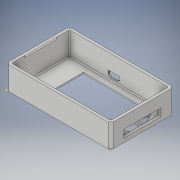
# Autodesk Inventor part: Top
Saved by Autodesk Inventor 2019 (Build 230136000, 136)
## iProperties
Created: 2021-04-22
Part Number: Top
Material: Všeobecné
Document SubType Name: Modeling
Designer: miko flosso
Density: 1 g/cm^3
Appearance: Výchozí
Author: miko flosso
Autodesk Inventor part; units mm, degrees
sketch "Náčrt1" plane through (0, 0, 0) normal (0, 1, 0) x (-1, 0, 0)
  line L0 (0, 0) -> (-81, 0)
  line L1 (-81, 0) -> (-81, -49)
  line L2 (-81, -49) -> (0, -49)
  line L3 (0, -49) -> (0, 0)
  dimension "d0" = 81
  dimension "d1" = 49
  constraints: 8 end point, 2 parallel, 1 horizontal, 1 perpendicular
  measures "d0" distance of L2.end L1.end
  measures "d1" distance of L1.end L0.end
extrude "Vysunutí1" add sketch "Náčrt1" along normal blind 20
chamfer "Zkosení1" distance 2 angle 45 8 edges at (40.5, 0, -49) (81, 0, -24.5) (81, 10, -49) (0, 10, -49) (40.5, 0, 0) (0, 0, -24.5) (81, 10, 0) (0, 10, 0)
shell "Skořepina1" thickness 2 removed faces 1 at (53.3333, 20, -16.3333)
sketch "Náčrt2" plane through (79, 2.8284, -46.1716) normal (-1, 0, 0) x (0, 0, 1)
  line L0 (9.1716, 17.1716) -> (34.1716, 17.1716)
  line L1 (34.1716, 17.1716) -> (34.1716, 15.6716)
  line L2 (34.1716, 15.6716) -> (9.1716, 15.6716)
  line L3 (9.1716, 15.6716) -> (9.1716, 17.1716)
  line L4 (0, 17.1716) -> (43.3431, 17.1716) projected
  point P0 (46.1716, -2.8284)
  point P1 (-0.8284, 17.1716)
  dimension "d8" = 25
  dimension "d9" = 1.5
  dimension "d11" = 10
  constraints: 8 end point, 2 parallel, 1 collinear, 1 horizontal, 1 perpendicular
  measures "d8" distance of L1.end L2.end
  measures "d9" distance of L0.end L1.end
  measures "d11" distance from line of point (-0.828, 17.172) L3
extrude "Vysunutí2" add sketch "Náčrt2" along normal blind 5 draft -45
ref_plane "Pracovní rovina1" through (40.5, 2.8284, -46.1716) normal (-1, 0, 0) x (0, 0, 1)
mirror "Zrcadlit1" about plane through (40.5, 2.8284, -46.1716) normal (-1, 0, 0) of "Vysunutí2"
sketch "Náčrt3" plane through (81, 2, -47) normal (1, 0, 0) x (0, 0, -1)
  line L0 (-8, 3) -> (-37, 3)
  line L1 (-37, 3) -> (-37, 9)
  line L2 (-37, 9) -> (-8, 9)
  line L3 (-8, 9) -> (-8, 3)
  line L4 (-45, -2) -> (0, -2) projected
  line L5 (2, 0) -> (2, 18) projected
  point P0 (-47, -2)
  dimension "d14" = 29
  dimension "d15" = 6
  dimension "d16" = 5
  dimension "d17" = 10
  constraints: 8 end point, 2 parallel, 1 horizontal, 1 perpendicular
  measures "d14" distance of L1.end L2.end
  measures "d15" distance of L0.end L1.end
  measures "d16" distance between parallel lines of L0 L4
  measures "d17" distance between parallel lines of L3 L5
extrude "Vysunutí3" cut sketch "Náčrt3" against normal blind 2.5
sketch "Náčrt4" plane through (79, 2.8284, -46.1716) normal (-1, 0, 0) x (0, 0, 1)
  line L0 (7.1716, 8.1716) -> (7.1716, 2.1716) projected
  line L1 (7.1716, 2.8716) -> (6.1716, 2.8716)
  line L2 (6.1716, 2.8716) -> (6.1716, 7.4716)
  line L3 (6.1716, 7.4716) -> (7.1716, 7.4716)
  line L4 (7.1716, 7.4716) -> (7.1716, 2.8716)
  line L5 (7.1716, 8.1716) -> (36.1716, 8.1716) projected
  point P0 (46.1716, -2.8284)
  dimension "d20" = 1
  dimension "d21" = 4.6
  dimension "d22" = 0.7
  constraints: 8 end point, 2 parallel, 1 horizontal, 1 perpendicular, 1 point on line
  measures "d20" distance of L2.end L3.end
  measures "d21" distance of L1.end L2.end
  measures "d22" distance between parallel lines of L3 L5
extrude "Vysunutí4" add sketch "Náčrt4" along normal blind 0.6
ref_plane "Pracovní rovina2" through (81, 5, -24.5) normal (0, 0, -1) x (-1, 0, 0)
sketch "Náčrt5" plane through (81, 5, -39) normal (0, 0, 1) x (1, 0, 0)
  line L0 (-2.6, 0.7) -> (-2.6, 5.3) projected
  line L1 (-2.6, 5.3) -> (-2, 5.3)
  line L2 (-2, 5.3) -> (-2, 0.7)
  line L3 (-2, 0.7) -> (-2.6, 0.7)
  line L4 (-2.6, 0.7) -> (-2.6, 5.3)
  point P0 (-81, -5)
  constraints: 8 end point, 2 parallel, 1 horizontal, 1 perpendicular
extrude "Vysunutí5" add sketch "Náčrt5" along normal blind 1.5 draft -45
mirror "Zrcadlit2" about plane through (81, 5, -24.5) normal (0, 0, -1) of "Vysunutí4", "Vysunutí5"
sketch "Náčrt6" plane through (0, 0, 0) normal (0, -1, 0) x (1, 0, 0)
  line L0 (63, -7) -> (18, -7)
  line L1 (18, -7) -> (18, -42)
  line L2 (18, -42) -> (63, -42)
  line L3 (63, -42) -> (63, -7)
  line L4 (0, -2) -> (0, -47) projected
  line L5 (2, -47) -> (2, -2) projected
  line L6 (79, -47) -> (2, -47) projected
  point P0 (0, 0)
  dimension "d27" = 45
  dimension "d28" = 35
  dimension "d30" = 16
  constraints: 8 end point, 2 parallel, 1 horizontal, 1 perpendicular
  measures "d27" distance of L2.end L1.end
  measures "d28" distance of L1.end L0.end
  measures "d30" distance between parallel lines of L5 L1
extrude "Vysunutí6" cut sketch "Náčrt6" against normal blind 2.5
sketch "Náčrt7" plane through (0, 0, 0) normal (0, -1, 0) x (1, 0, 0)
  line L0 (64, -43) -> (17, -43)
  line L1 (17, -43) -> (17, -6)
  line L2 (17, -6) -> (64, -6)
  line L3 (64, -6) -> (64, -43)
  line L4 (63, -7) -> (63, -42) projected
  line L5 (63, -42) -> (18, -42) projected
  line L6 (18, -42) -> (18, -7) projected
  point P0 (0, 0)
  dimension "d34" = 47
  dimension "d35" = 37
  dimension "d37" = 1
  dimension "d95" = 1
  constraints: 8 end point, 2 parallel, 1 horizontal, 1 perpendicular
  measures "d34" distance of L1.end L2.end
  measures "d35" distance of L0.end L1.end
  measures "d37" distance between parallel lines of L0 L5
  measures "d95" distance between parallel lines of L6 L1
extrude "Vysunutí7" cut sketch "Náčrt7" against normal blind 1
sketch "Náčrt8" plane through (0, 0, 0) normal (0, -1, 0) x (1, 0, 0)
  line L0 (69, -29) -> (75, -29)
  line L1 (75, -29) -> (75, -20)
  line L2 (75, -20) -> (69, -20)
  line L3 (69, -20) -> (69, -29)
  line L4 (64, -6) -> (64, -43) projected
  line L5 (2, -2) -> (79, -2) projected
  line L6 (68.5, -32) -> (75.5, -32)
  line L7 (68.5, -32) -> (72, -40)
  line L8 (75.5, -32) -> (72, -40)
  point P0 (0, 0)
  dimension "d40" = 6
  dimension "d41" = 9
  dimension "d42" = 5
  dimension "d43" = 18
  dimension "d45" = 3
  dimension "d46" = 7
  constraints: 14 end point, 2 horizontal, 2 parallel, 1 perpendicular
  measures "d40" distance of L2.end L1.end
  measures "d41" distance of L1.end L0.end
  measures "d42" distance between parallel lines of L4 L3
  measures "d43" distance between parallel lines of L5 L2
  measures "d45" distance between parallel lines of L0 L6
  measures "d46" distance of L6.start L6.end
extrude "Vysunutí8" cut sketch "Náčrt8" against normal blind 2.5 contours L6 L8 L7
chamfer "Zkosení2" distance 1 angle 45 2 edges at (75.5, 1, -32) (68.5, 1, -32)
sketch "Náčrt9" plane through (0, 0, 0) normal (0, -1, 0) x (1, 0, 0)
  line L0 (69, -29) -> (75, -29)
  line L1 (75, -29) -> (75, -20)
  line L2 (75, -20) -> (69, -20)
  line L3 (69, -20) -> (69, -29)
  line L4 (64, -6) -> (64, -43) projected
  line L5 (2, -2) -> (79, -2) projected
  point P0 (0, 0)
  dimension "d54" = 6
  dimension "d55" = 9
  dimension "d56" = 5
  dimension "d57" = 18
  constraints: 8 end point, 2 parallel, 1 horizontal, 1 perpendicular
  measures "d54" distance of L2.end L1.end
  measures "d55" distance of L1.end L0.end
  measures "d56" distance between parallel lines of L4 L3
  measures "d57" distance between parallel lines of L5 L2
extrude "Vysunutí9" cut sketch "Náčrt9" against normal blind 2.5
chamfer "Zkosení3" distance 1 angle 45 4 edges at (75, 1, -29) (69, 1, -29) (69, 1, -20) (75, 1, -20)
sketch "Náčrt10" plane through (2.8284, 2, -2.8284) normal (0, 1, 0) x (1, 0, 0)
  point P0 (-2.8284, -2.8284)
chamfer "Zkosení4" distance 1 angle 45 1 edges at (72, 1, -40)
ref_plane "Pracovní rovina3" through (78.1716, 20, -24.5) normal (0, 0, -1) x (-1, 0, 0)
mirror "Zrcadlit4" about plane through (78.1716, 20, -24.5) normal (0, 0, -1) of "Vysunutí8", "Zkosení2"
chamfer "Zkosení5" distance 1 angle 45 1 edges at (72, 1, -9)
sketch "Náčrt11" plane through (2.8284, 2, -2.8284) normal (0, 1, 0) x (1, 0, 0)
  line L0 (64.5716, 28.3216) -> (73.7716, 28.3216)
  line L1 (71.6716, 29.1716) -> (66.6716, 29.1716) projected
  line L2 (73.7716, 28.3216) -> (69.1716, 38.5216)
  line L3 (64.5716, 28.3216) -> (69.1716, 38.5216)
  point P0 (-2.8284, -2.8284)
  point P1 (75.3431, 29.1716)
  dimension "d73" = 0.85
  constraints: 6 end point, 1 horizontal
  measures "d73" distance between parallel lines of L0 L1
extrude "Vysunutí10" cut sketch "Náčrt11" against normal blind 1
chamfer "Zkosení6" distance 1.1 angle 45 3 edges at (76.6, 1.5, -31.15) (67.4, 1.5, -31.15) (72, 1.5, -41.35)
mirror "Zrcadlit5" about plane through (78.1716, 20, -24.5) normal (0, 0, -1) of "Vysunutí10", "Zkosení6"
sketch "Náčrt12" plane through (2.8284, 2, -2.8284) normal (0, 1, 0) x (1, 0, 0)
  line L0 (73.2716, 27.2716) -> (65.0716, 27.2716)
  line L1 (65.0716, 27.2716) -> (65.0716, 16.0716)
  line L2 (65.0716, 16.0716) -> (73.2716, 16.0716)
  line L3 (73.2716, 16.0716) -> (73.2716, 27.2716)
  line L4 (66.1716, 18.1716) -> (66.1716, 25.1716) projected
  line L5 (71.1716, 17.1716) -> (67.1716, 17.1716) projected
  point P0 (-2.8284, -2.8284)
  point P1 (75.3431, 17.1716)
  dimension "d80" = 8.2
  dimension "d81" = 11.2
  dimension "d82" = 1.1
  dimension "d83" = 1.1
  constraints: 8 end point, 2 parallel, 1 horizontal, 1 perpendicular
  measures "d80" distance of L2.end L1.end
  measures "d81" distance of L1.end L0.end
  measures "d82" distance between parallel lines of L4 L1
  measures "d83" distance between parallel lines of L5 L2
extrude "Vysunutí11" cut sketch "Náčrt12" against normal blind 1
chamfer "Zkosení7" distance 1.1 angle 45 4 edges at (76.1, 1.5, -18.9) (67.9, 1.5, -18.9) (67.9, 1.5, -30.1) (76.1, 1.5, -30.1)
sketch "Náčrt13" plane through (79, 2, -49) normal (0, 0, -1) x (-1, 0, 0)
  line L0 (47, 2) -> (38, 2)
  line L1 (38, 2) -> (38, 6)
  line L2 (38, 6) -> (47, 6)
  line L3 (47, 6) -> (47, 2)
  line L4 (0, -2) -> (77, -2) projected
  point P0 (79, -2)
  point P1 (61, -1)
  dimension "d89" = 9
  dimension "d90" = 4
  dimension "d91" = 14
  dimension "d92" = 4
  constraints: 8 end point, 2 parallel, 1 horizontal, 1 perpendicular
  measures "d89" distance of L1.end L2.end
  measures "d90" distance of L0.end L1.end
  measures "d91" distance from line of point (61, -1) L3
  measures "d92" distance between parallel lines of L4 L0
extrude "Vysunutí12" cut sketch "Náčrt13" against normal blind 2.5
chamfer "Zkosení8" distance 2 angle 30 2 edges at (32, 4, -48) (41, 4, -48) measured on face at (32.5, 4, -48) measured on face at (40.5, 4, -48)
sketch "Náčrt14" plane through (79, 2, -49) normal (0, 0, -1) x (-1, 0, 0)
  line L0 (47.5, 7) -> (37.5, 7)
  line L1 (37.5, 7) -> (37.5, 1)
  line L2 (37.5, 1) -> (47.5, 1)
  line L3 (47.5, 1) -> (47.5, 7)
  line L4 (47.5, 7) -> (37.5, 1) construction
  line L5 (37.5, 7) -> (47.5, 1) construction
  line L6 (45, 2) -> (40, 2) projected
  line L7 (38, 3.1547) -> (38, 6) projected
  point P0 (79, -2)
  point P1 (42.5, 4)
  dimension "d99" = 10
  dimension "d100" = 6
  dimension "d101" = 1
  dimension "d102" = 0.5
  constraints: 12 end point, 2 midpoint, 2 parallel, 1 horizontal, 1 perpendicular
  measures "d99" distance of L2.end L1.end
  measures "d100" distance of L1.end L0.end
  measures "d101" distance between parallel lines of L6 L2
  measures "d102" distance between parallel lines of L1 L7
extrude "Vysunutí13" cut sketch "Náčrt14" against normal blind 1
chamfer "Zkosení9" distance 1 angle 45 4 edges at (41.5, 3, -48.5) (31.5, 3, -48.5) (41.5, 9, -48.5) (31.5, 9, -48.5)
chamfer "Zkosení10" distance 0.5 angle 45 2 edges at (41, 8, -47.5) (32, 8, -47.5)
